Autodesk Fusion 360 part; units mm, degrees
note: some values were not read from the file. Chosen so that the rebuilt part matches the saved one: a direction. Set by a fixed rule: which sketch regions a step uses; which face or edge a step refers to.
(part 2 of 6)
  spline S261 degree 3 poles (85.6721, -57.6527) (85.6866, -57.6527) (85.6985, -57.6408) (85.6985, -57.6263) knots 0 0 0 0 1 1 1 1
  line L291 (85.6985, -57.6263) -> (85.6985, -56.0388)
  spline S262 degree 3 poles (85.6985, -56.0388) (85.6985, -56.0242) (85.6866, -56.0123) (85.6721, -56.0123) knots 0 0 0 0 1 1 1 1
  line L292 (85.6721, -56.0123) -> (84.9048, -56.0123)
  spline S263 degree 3 poles (84.9048, -56.0123) (84.8783, -56.0123) (84.9048, -56.0388) (84.9048, -56.0123) knots 0 0 0 0 1 1 1 1
  line L293 (84.9048, -56.0123) -> (84.9048, -54.4777)
  spline S264 degree 3 poles (84.9048, -54.4777) (84.9048, -54.4513) (84.8783, -54.4777) (84.9048, -54.4777) knots 0 0 0 0 1 1 1 1
  line L294 (84.9048, -54.4777) -> (85.6721, -54.4777)
  spline S265 degree 3 poles (85.6721, -54.4777) (85.6866, -54.4777) (85.6985, -54.4658) (85.6985, -54.4513) knots 0 0 0 0 1 1 1 1
  line L295 (85.6985, -54.4513) -> (85.6985, -52.8638)
  spline S266 degree 3 poles (85.6985, -52.8638) (85.6985, -52.8492) (85.6866, -52.8373) (85.6721, -52.8373) knots 0 0 0 0 1 1 1 1
  line L296 (85.6721, -52.8373) -> (84.9048, -52.8373)
  spline S267 degree 3 poles (84.9048, -52.8373) (84.8783, -52.8373) (84.9048, -52.8638) (84.9048, -52.8373) knots 0 0 0 0 1 1 1 1
  line L297 (84.9048, -52.8373) -> (84.9048, -51.3027)
  spline S268 degree 3 poles (84.9048, -51.3027) (84.9048, -51.2763) (84.8783, -51.3027) (84.9048, -51.3027) knots 0 0 0 0 1 1 1 1
  line L298 (84.9048, -51.3027) -> (85.6721, -51.3027)
  spline S269 degree 3 poles (85.6721, -51.3027) (85.6866, -51.3027) (85.6985, -51.2908) (85.6985, -51.2763) knots 0 0 0 0 1 1 1 1
  line L299 (85.6985, -51.2763) -> (85.6985, -49.6888)
  spline S270 degree 3 poles (85.6985, -49.6888) (85.6985, -49.6742) (85.6866, -49.6623) (85.6721, -49.6623) knots 0 0 0 0 1 1 1 1
  line L300 (85.6721, -49.6623) -> (84.9048, -49.6623)
  spline S271 degree 3 poles (84.9048, -49.6623) (84.8783, -49.6623) (84.9048, -49.6888) (84.9048, -49.6623) knots 0 0 0 0 1 1 1 1
  line L301 (84.9048, -49.6623) -> (84.9048, -48.1277)
  spline S272 degree 3 poles (84.9048, -48.1277) (84.9048, -48.1013) (84.8783, -48.1277) (84.9048, -48.1277) knots 0 0 0 0 1 1 1 1
  line L302 (84.9048, -48.1277) -> (85.6721, -48.1277)
  spline S273 degree 3 poles (85.6721, -48.1277) (85.6866, -48.1277) (85.6985, -48.1158) (85.6985, -48.1013) knots 0 0 0 0 1 1 1 1
  line L303 (85.6985, -48.1013) -> (85.6985, -46.5138)
  spline S274 degree 3 poles (85.6985, -46.5138) (85.6985, -46.4992) (85.6866, -46.4873) (85.6721, -46.4873) knots 0 0 0 0 1 1 1 1
  line L304 (85.6721, -46.4873) -> (84.9048, -46.4873)
  spline S275 degree 3 poles (84.9048, -46.4873) (84.8783, -46.4873) (84.9048, -46.5138) (84.9048, -46.4873) knots 0 0 0 0 1 1 1 1
  line L305 (84.9048, -46.4873) -> (84.9048, -44.9527)
  spline S276 degree 3 poles (84.9048, -44.9527) (84.9048, -44.9263) (84.8783, -44.9527) (84.9048, -44.9527) knots 0 0 0 0 1 1 1 1
  line L306 (84.9048, -44.9527) -> (85.6721, -44.9527)
  spline S277 degree 3 poles (85.6721, -44.9527) (85.6866, -44.9527) (85.6985, -44.9408) (85.6985, -44.9263) knots 0 0 0 0 1 1 1 1
  line L307 (85.6985, -44.9263) -> (85.6985, -43.3388)
  spline S278 degree 3 poles (85.6985, -43.3388) (85.6985, -43.3242) (85.6866, -43.3123) (85.6721, -43.3123) knots 0 0 0 0 1 1 1 1
  line L308 (85.6721, -43.3123) -> (84.9048, -43.3123)
  spline S279 degree 3 poles (84.9048, -43.3123) (84.8783, -43.3123) (84.9048, -43.3388) (84.9048, -43.3123) knots 0 0 0 0 1 1 1 1
  line L309 (84.9048, -43.3123) -> (84.9048, -42.5715)
  spline S280 degree 3 poles (84.9048, -42.5715) (84.9048, -42.545) (84.8783, -42.5715) (84.9048, -42.5715) knots 0 0 0 0 1 1 1 1
  line L310 (84.9048, -42.5715) -> (85.6721, -42.5715)
  spline S281 degree 3 poles (85.6721, -42.5715) (85.6866, -42.5715) (85.6985, -42.5596) (85.6985, -42.545) knots 0 0 0 0 1 1 1 1
  spline S282 degree 3 poles (85.6985, -42.545) (85.6985, -40.5432) (85.1718, -38.5768) (84.1708, -36.8432) knots 0 0 0 0 1 1 1 1
  spline S283 degree 3 poles (84.1708, -36.8432) (83.1699, -35.1097) (81.7303, -33.6701) (79.9968, -32.6692) knots 0 0 0 0 1 1 1 1
  spline S284 degree 3 poles (79.9968, -32.6692) (78.2632, -31.6682) (76.2968, -31.1415) (74.295, -31.1415) knots 0 0 0 0 1 1 1 1
  line L311 (74.295, -31.1415) -> (45.1908, -31.1415)
  spline S285 degree 3 poles (45.1908, -31.1415) (45.1763, -31.1415) (45.1644, -31.1534) (45.1644, -31.1679) knots 0 0 0 0 1 1 1 1
  line L312 (45.1644, -31.1679) -> (45.1644, -31.9617)
  line L313 (45.1644, -31.9617) -> (45.1644, -33.2581)
  spline S286 degree 3 poles (45.1644, -33.2581) (45.1644, -33.2846) (45.1908, -33.2581) (45.1644, -33.2581) knots 0 0 0 0 1 1 1 1
  line L314 (45.1644, -33.2581) -> (44.3971, -33.2581)
  spline S287 degree 3 poles (44.3971, -33.2581) (44.3825, -33.2581) (44.3706, -33.27) (44.3706, -33.2846) knots 0 0 0 0 1 1 1 1
  line L315 (44.3706, -33.2846) -> (44.3706, -34.8721)
  spline S288 degree 3 poles (44.3706, -34.8721) (44.3706, -34.8866) (44.3825, -34.8985) (44.3971, -34.8985) knots 0 0 0 0 1 1 1 1
  line L316 (44.3971, -34.8985) -> (45.1644, -34.8985)
  spline S289 degree 3 poles (45.1644, -34.8985) (45.1908, -34.8985) (45.1644, -34.8721) (45.1644, -34.8985) knots 0 0 0 0 1 1 1 1
  line L317 (45.1644, -34.8985) -> (45.1644, -36.4331)
  spline S290 degree 3 poles (45.1644, -36.4331) (45.1644, -36.4596) (45.1908, -36.4331) (45.1644, -36.4331) knots 0 0 0 0 1 1 1 1
  line L318 (45.1644, -36.4331) -> (44.3971, -36.4331)
  spline S291 degree 3 poles (44.3971, -36.4331) (44.3825, -36.4331) (44.3706, -36.445) (44.3706, -36.4596) knots 0 0 0 0 1 1 1 1
  line L319 (44.3706, -36.4596) -> (44.3706, -38.0471)
  spline S292 degree 3 poles (44.3706, -38.0471) (44.3706, -38.0616) (44.3825, -38.0735) (44.3971, -38.0735) knots 0 0 0 0 1 1 1 1
  line L320 (44.3971, -38.0735) -> (45.1644, -38.0735)
  spline S293 degree 3 poles (45.1644, -38.0735) (45.1908, -38.0735) (45.1644, -38.0471) (45.1644, -38.0735) knots 0 0 0 0 1 1 1 1
  line L321 (45.1644, -38.0735) -> (45.1644, -39.6081)
  spline S294 degree 3 poles (45.1644, -39.6081) (45.1644, -39.6346) (45.1908, -39.6081) (45.1644, -39.6081) knots 0 0 0 0 1 1 1 1
  line L322 (45.1644, -39.6081) -> (44.3971, -39.6081)
  spline S295 degree 3 poles (44.3971, -39.6081) (44.3825, -39.6081) (44.3706, -39.62) (44.3706, -39.6346) knots 0 0 0 0 1 1 1 1
  line L323 (44.3706, -39.6346) -> (44.3706, -41.2221)
  spline S296 degree 3 poles (44.3706, -41.2221) (44.3706, -41.2366) (44.3825, -41.2485) (44.3971, -41.2485) knots 0 0 0 0 1 1 1 1
  line L324 (44.3971, -41.2485) -> (45.1644, -41.2485)
  spline S297 degree 3 poles (45.1644, -41.2485) (45.1908, -41.2485) (45.1644, -41.2221) (45.1644, -41.2485) knots 0 0 0 0 1 1 1 1
  line L325 (45.1644, -41.2485) -> (45.1644, -42.7831)
  spline S298 degree 3 poles (45.1644, -42.7831) (45.1644, -42.8096) (45.1908, -42.7831) (45.1644, -42.7831) knots 0 0 0 0 1 1 1 1
  line L326 (45.1644, -42.7831) -> (44.3971, -42.7831)
  spline S299 degree 3 poles (44.3971, -42.7831) (44.3825, -42.7831) (44.3706, -42.795) (44.3706, -42.8096) knots 0 0 0 0 1 1 1 1
  line L327 (44.3706, -42.8096) -> (44.3706, -44.3971)
  spline S300 degree 3 poles (44.3706, -44.3971) (44.3706, -44.4116) (44.3825, -44.4235) (44.3971, -44.4235) knots 0 0 0 0 1 1 1 1
  line L328 (44.3971, -44.4235) -> (45.1644, -44.4235)
  spline S301 degree 3 poles (45.1644, -44.4235) (45.1908, -44.4235) (45.1644, -44.3971) (45.1644, -44.4235) knots 0 0 0 0 1 1 1 1
  line L329 (45.1644, -44.4235) -> (45.1644, -45.9581)
  spline S302 degree 3 poles (45.1644, -45.9581) (45.1644, -45.9846) (45.1908, -45.9581) (45.1644, -45.9581) knots 0 0 0 0 1 1 1 1
  line L330 (45.1644, -45.9581) -> (44.3971, -45.9581)
  spline S303 degree 3 poles (44.3971, -45.9581) (44.3825, -45.9581) (44.3706, -45.97) (44.3706, -45.9846) knots 0 0 0 0 1 1 1 1
  line L331 (44.3706, -45.9846) -> (44.3706, -47.5721)
  spline S304 degree 3 poles (44.3706, -47.5721) (44.3706, -47.5866) (44.3825, -47.5985) (44.3971, -47.5985) knots 0 0 0 0 1 1 1 1
  line L332 (44.3971, -47.5985) -> (45.1644, -47.5985)
  spline S305 degree 3 poles (45.1644, -47.5985) (45.1908, -47.5985) (45.1644, -47.5721) (45.1644, -47.5985) knots 0 0 0 0 1 1 1 1
  line L333 (45.1644, -47.5985) -> (45.1644, -49.1331)
  spline S306 degree 3 poles (45.1644, -49.1331) (45.1644, -49.1596) (45.1908, -49.1331) (45.1644, -49.1331) knots 0 0 0 0 1 1 1 1
  line L334 (45.1644, -49.1331) -> (44.3971, -49.1331)
  spline S307 degree 3 poles (44.3971, -49.1331) (44.3825, -49.1331) (44.3706, -49.145) (44.3706, -49.1596) knots 0 0 0 0 1 1 1 1
  line L335 (44.3706, -49.1596) -> (44.3706, -50.7471)
  spline S308 degree 3 poles (44.3706, -50.7471) (44.3706, -50.7616) (44.3825, -50.7735) (44.3971, -50.7735) knots 0 0 0 0 1 1 1 1
  line L336 (44.3971, -50.7735) -> (45.1644, -50.7735)
  spline S309 degree 3 poles (45.1644, -50.7735) (45.1908, -50.7735) (45.1644, -50.7471) (45.1644, -50.7735) knots 0 0 0 0 1 1 1 1
  line L337 (45.1644, -50.7735) -> (45.1644, -52.3081)
  spline S310 degree 3 poles (45.1644, -52.3081) (45.1644, -52.3346) (45.1908, -52.3081) (45.1644, -52.3081) knots 0 0 0 0 1 1 1 1
  line L338 (45.1644, -52.3081) -> (44.3971, -52.3081)
  spline S311 degree 3 poles (44.3971, -52.3081) (44.3825, -52.3081) (44.3706, -52.32) (44.3706, -52.3346) knots 0 0 0 0 1 1 1 1
  line L339 (44.3706, -52.3346) -> (44.3706, -53.9221)
  spline S312 degree 3 poles (44.3706, -53.9221) (44.3706, -53.9366) (44.3825, -53.9485) (44.3971, -53.9485) knots 0 0 0 0 1 1 1 1
  line L340 (44.3971, -53.9485) -> (45.1644, -53.9485)
  spline S313 degree 3 poles (45.1644, -53.9485) (45.1908, -53.9485) (45.1644, -53.9221) (45.1644, -53.9485) knots 0 0 0 0 1 1 1 1
  line L341 (45.1644, -53.9485) -> (45.1644, -55.4831)
  spline S314 degree 3 poles (45.1644, -55.4831) (45.1644, -55.5096) (45.1908, -55.4831) (45.1644, -55.4831) knots 0 0 0 0 1 1 1 1
  line L342 (45.1644, -55.4831) -> (44.3971, -55.4831)
  spline S315 degree 3 poles (44.3971, -55.4831) (44.3825, -55.4831) (44.3706, -55.495) (44.3706, -55.5096) knots 0 0 0 0 1 1 1 1
  line L343 (44.3706, -55.5096) -> (44.3706, -57.0971)
  spline S316 degree 3 poles (44.3706, -57.0971) (44.3706, -57.1116) (44.3825, -57.1235) (44.3971, -57.1235) knots 0 0 0 0 1 1 1 1
  line L344 (44.3971, -57.1235) -> (45.1644, -57.1235)
  spline S317 degree 3 poles (45.1644, -57.1235) (45.1908, -57.1235) (45.1644, -57.0971) (45.1644, -57.1235) knots 0 0 0 0 1 1 1 1
  line L345 (45.1644, -57.1235) -> (45.1644, -58.42)
  line L346 (86.9156, -58.4465) -> (88.2121, -58.4465)
  spline S318 degree 3 poles (88.2121, -58.4465) (88.2385, -58.4465) (88.2121, -58.42) (88.2121, -58.4465) knots 0 0 0 0 1 1 1 1
  line L347 (88.2121, -58.4465) -> (88.2121, -59.2138)
  spline S319 degree 3 poles (88.2121, -59.2138) (88.2121, -59.2283) (88.224, -59.2402) (88.2385, -59.2402) knots 0 0 0 0 1 1 1 1
  line L348 (88.2385, -59.2402) -> (89.826, -59.2402)
  spline S320 degree 3 poles (89.826, -59.2402) (89.8406, -59.2402) (89.8525, -59.2283) (89.8525, -59.2138) knots 0 0 0 0 1 1 1 1
  line L349 (89.8525, -59.2138) -> (89.8525, -58.4465)
  spline S321 degree 3 poles (89.8525, -58.4465) (89.8525, -58.42) (89.826, -58.4465) (89.8525, -58.4465) knots 0 0 0 0 1 1 1 1
  line L350 (89.8525, -58.4465) -> (91.3871, -58.4465)
  spline S322 degree 3 poles (91.3871, -58.4465) (91.4135, -58.4465) (91.3871, -58.42) (91.3871, -58.4465) knots 0 0 0 0 1 1 1 1
  line L351 (91.3871, -58.4465) -> (91.3871, -59.2138)
  spline S323 degree 3 poles (91.3871, -59.2138) (91.3871, -59.2283) (91.399, -59.2402) (91.4135, -59.2402) knots 0 0 0 0 1 1 1 1
  line L352 (91.4135, -59.2402) -> (93.001, -59.2402)
  spline S324 degree 3 poles (93.001, -59.2402) (93.0156, -59.2402) (93.0275, -59.2283) (93.0275, -59.2138) knots 0 0 0 0 1 1 1 1
  line L353 (93.0275, -59.2138) -> (93.0275, -58.4465)
  spline S325 degree 3 poles (93.0275, -58.4465) (93.0275, -58.42) (93.001, -58.4465) (93.0275, -58.4465) knots 0 0 0 0 1 1 1 1
  line L354 (93.0275, -58.4465) -> (94.5621, -58.4465)
  spline S326 degree 3 poles (94.5621, -58.4465) (94.5885, -58.4465) (94.5621, -58.42) (94.5621, -58.4465) knots 0 0 0 0 1 1 1 1
  line L355 (94.5621, -58.4465) -> (94.5621, -59.2138)
  spline S327 degree 3 poles (94.5621, -59.2138) (94.5621, -59.2283) (94.574, -59.2402) (94.5885, -59.2402) knots 0 0 0 0 1 1 1 1
  line L356 (94.5885, -59.2402) -> (96.176, -59.2402)
  spline S328 degree 3 poles (96.176, -59.2402) (96.1906, -59.2402) (96.2025, -59.2283) (96.2025, -59.2138) knots 0 0 0 0 1 1 1 1
  line L357 (96.2025, -59.2138) -> (96.2025, -58.4465)
  spline S329 degree 3 poles (96.2025, -58.4465) (96.2025, -58.42) (96.176, -58.4465) (96.2025, -58.4465) knots 0 0 0 0 1 1 1 1
  line L358 (96.2025, -58.4465) -> (97.7371, -58.4465)
  spline S330 degree 3 poles (97.7371, -58.4465) (97.7635, -58.4465) (97.7371, -58.42) (97.7371, -58.4465) knots 0 0 0 0 1 1 1 1
  line L359 (97.7371, -58.4465) -> (97.7371, -59.2138)
  spline S331 degree 3 poles (97.7371, -59.2138) (97.7371, -59.2283) (97.749, -59.2402) (97.7635, -59.2402) knots 0 0 0 0 1 1 1 1
  line L360 (97.7635, -59.2402) -> (99.351, -59.2402)
  spline S332 degree 3 poles (99.351, -59.2402) (99.3656, -59.2402) (99.3775, -59.2283) (99.3775, -59.2138) knots 0 0 0 0 1 1 1 1
  line L361 (99.3775, -59.2138) -> (99.3775, -58.4465)
  spline S333 degree 3 poles (99.3775, -58.4465) (99.3775, -58.42) (99.351, -58.4465) (99.3775, -58.4465) knots 0 0 0 0 1 1 1 1
  line L362 (99.3775, -58.4465) -> (100.9121, -58.4465)
  spline S334 degree 3 poles (100.9121, -58.4465) (100.9385, -58.4465) (100.9121, -58.42) (100.9121, -58.4465) knots 0 0 0 0 1 1 1 1
  line L363 (100.9121, -58.4465) -> (100.9121, -59.2138)
  spline S335 degree 3 poles (100.9121, -59.2138) (100.9121, -59.2283) (100.924, -59.2402) (100.9385, -59.2402) knots 0 0 0 0 1 1 1 1
  line L364 (100.9385, -59.2402) -> (102.526, -59.2402)
  spline S336 degree 3 poles (102.526, -59.2402) (102.5406, -59.2402) (102.5525, -59.2283) (102.5525, -59.2138) knots 0 0 0 0 1 1 1 1
  line L365 (102.5525, -59.2138) -> (102.5525, -58.4465)
  spline S337 degree 3 poles (102.5525, -58.4465) (102.5525, -58.42) (102.526, -58.4465) (102.5525, -58.4465) knots 0 0 0 0 1 1 1 1
  line L366 (102.5525, -58.4465) -> (104.0871, -58.4465)
  spline S338 degree 3 poles (104.0871, -58.4465) (104.1135, -58.4465) (104.0871, -58.42) (104.0871, -58.4465) knots 0 0 0 0 1 1 1 1
  line L367 (104.0871, -58.4465) -> (104.0871, -59.2138)
  spline S339 degree 3 poles (104.0871, -59.2138) (104.0871, -59.2283) (104.099, -59.2402) (104.1135, -59.2402) knots 0 0 0 0 1 1 1 1
  line L368 (104.1135, -59.2402) -> (105.701, -59.2402)
  spline S340 degree 3 poles (105.701, -59.2402) (105.7156, -59.2402) (105.7275, -59.2283) (105.7275, -59.2138) knots 0 0 0 0 1 1 1 1
  line L369 (105.7275, -59.2138) -> (105.7275, -58.4465)
  spline S341 degree 3 poles (105.7275, -58.4465) (105.7275, -58.42) (105.701, -58.4465) (105.7275, -58.4465) knots 0 0 0 0 1 1 1 1
  line L370 (105.7275, -58.4465) -> (107.2621, -58.4465)
  spline S342 degree 3 poles (107.2621, -58.4465) (107.2885, -58.4465) (107.2621, -58.42) (107.2621, -58.4465) knots 0 0 0 0 1 1 1 1
  line L371 (107.2621, -58.4465) -> (107.2621, -59.2138)
  spline S343 degree 3 poles (107.2621, -59.2138) (107.2621, -59.2283) (107.274, -59.2402) (107.2885, -59.2402) knots 0 0 0 0 1 1 1 1
  line L372 (107.2885, -59.2402) -> (108.876, -59.2402)
  spline S344 degree 3 poles (108.876, -59.2402) (108.8906, -59.2402) (108.9025, -59.2283) (108.9025, -59.2138) knots 0 0 0 0 1 1 1 1
  line L373 (108.9025, -59.2138) -> (108.9025, -58.4465)
  spline S345 degree 3 poles (108.9025, -58.4465) (108.9025, -58.42) (108.876, -58.4465) (108.9025, -58.4465) knots 0 0 0 0 1 1 1 1
  line L374 (108.9025, -58.4465) -> (110.4371, -58.4465)
  spline S346 degree 3 poles (110.4371, -58.4465) (110.4635, -58.4465) (110.4371, -58.42) (110.4371, -58.4465) knots 0 0 0 0 1 1 1 1
  line L375 (110.4371, -58.4465) -> (110.4371, -59.2138)
  spline S347 degree 3 poles (110.4371, -59.2138) (110.4371, -59.2283) (110.449, -59.2402) (110.4635, -59.2402) knots 0 0 0 0 1 1 1 1
  line L376 (110.4635, -59.2402) -> (112.051, -59.2402)
  spline S348 degree 3 poles (112.051, -59.2402) (112.0656, -59.2402) (112.0775, -59.2283) (112.0775, -59.2138) knots 0 0 0 0 1 1 1 1
  line L377 (112.0775, -59.2138) -> (112.0775, -58.4465)
  spline S349 degree 3 poles (112.0775, -58.4465) (112.0775, -58.42) (112.051, -58.4465) (112.0775, -58.4465) knots 0 0 0 0 1 1 1 1
  line L378 (112.0775, -58.4465) -> (113.374, -58.4465)
  line L379 (113.374, -58.4465) -> (114.1677, -58.4465)
  spline S350 degree 3 poles (114.1677, -58.4465) (114.1823, -58.4465) (114.1942, -58.4346) (114.1942, -58.42) knots 0 0 0 0 1 1 1 1
  line L380 (114.1942, -58.42) -> (114.1942, -57.0971)
  spline S351 degree 3 poles (114.1942, -57.0971) (114.1942, -57.0825) (114.1823, -57.0706) (114.1677, -57.0706) knots 0 0 0 0 1 1 1 1
  line L381 (114.1677, -57.0706) -> (113.4004, -57.0706)
  spline S352 degree 3 poles (113.4004, -57.0706) (113.374, -57.0706) (113.4004, -57.0971) (113.4004, -57.0706) knots 0 0 0 0 1 1 1 1
  line L382 (113.4004, -57.0706) -> (113.4004, -55.536)
  spline S353 degree 3 poles (113.4004, -55.536) (113.4004, -55.5096) (113.374, -55.536) (113.4004, -55.536) knots 0 0 0 0 1 1 1 1
  line L383 (113.4004, -55.536) -> (114.1677, -55.536)
  spline S354 degree 3 poles (114.1677, -55.536) (114.1823, -55.536) (114.1942, -55.5241) (114.1942, -55.5096) knots 0 0 0 0 1 1 1 1
  line L384 (114.1942, -55.5096) -> (114.1942, -53.9221)
  spline S355 degree 3 poles (114.1942, -53.9221) (114.1942, -53.9075) (114.1823, -53.8956) (114.1677, -53.8956) knots 0 0 0 0 1 1 1 1
  line L385 (114.1677, -53.8956) -> (113.4004, -53.8956)
  spline S356 degree 3 poles (113.4004, -53.8956) (113.374, -53.8956) (113.4004, -53.9221) (113.4004, -53.8956) knots 0 0 0 0 1 1 1 1
  line L386 (113.4004, -53.8956) -> (113.4004, -52.361)
  spline S357 degree 3 poles (113.4004, -52.361) (113.4004, -52.3346) (113.374, -52.361) (113.4004, -52.361) knots 0 0 0 0 1 1 1 1
  line L387 (113.4004, -52.361) -> (114.1677, -52.361)
  spline S358 degree 3 poles (114.1677, -52.361) (114.1823, -52.361) (114.1942, -52.3491) (114.1942, -52.3346) knots 0 0 0 0 1 1 1 1
  line L388 (114.1942, -52.3346) -> (114.1942, -50.7471)
  spline S359 degree 3 poles (114.1942, -50.7471) (114.1942, -50.7325) (114.1823, -50.7206) (114.1677, -50.7206) knots 0 0 0 0 1 1 1 1
  line L389 (114.1677, -50.7206) -> (113.4004, -50.7206)
  spline S360 degree 3 poles (113.4004, -50.7206) (113.374, -50.7206) (113.4004, -50.7471) (113.4004, -50.7206) knots 0 0 0 0 1 1 1 1
  line L390 (113.4004, -50.7206) -> (113.4004, -49.186)
  spline S361 degree 3 poles (113.4004, -49.186) (113.4004, -49.1596) (113.374, -49.186) (113.4004, -49.186) knots 0 0 0 0 1 1 1 1
  line L391 (113.4004, -49.186) -> (114.1677, -49.186)
  spline S362 degree 3 poles (114.1677, -49.186) (114.1823, -49.186) (114.1942, -49.1741) (114.1942, -49.1596) knots 0 0 0 0 1 1 1 1
  line L392 (114.1942, -49.1596) -> (114.1942, -47.5721)
  spline S363 degree 3 poles (114.1942, -47.5721) (114.1942, -47.5575) (114.1823, -47.5456) (114.1677, -47.5456) knots 0 0 0 0 1 1 1 1
  line L393 (114.1677, -47.5456) -> (113.4004, -47.5456)
  spline S364 degree 3 poles (113.4004, -47.5456) (113.374, -47.5456) (113.4004, -47.5721) (113.4004, -47.5456) knots 0 0 0 0 1 1 1 1
  line L394 (113.4004, -47.5456) -> (113.4004, -46.011)
  spline S365 degree 3 poles (113.4004, -46.011) (113.4004, -45.9846) (113.374, -46.011) (113.4004, -46.011) knots 0 0 0 0 1 1 1 1
  line L395 (113.4004, -46.011) -> (114.1677, -46.011)
  spline S366 degree 3 poles (114.1677, -46.011) (114.1823, -46.011) (114.1942, -45.9991) (114.1942, -45.9846) knots 0 0 0 0 1 1 1 1
  line L396 (114.1942, -45.9846) -> (114.1942, -44.3971)
  spline S367 degree 3 poles (114.1942, -44.3971) (114.1942, -44.3825) (114.1823, -44.3706) (114.1677, -44.3706) knots 0 0 0 0 1 1 1 1
  line L397 (114.1677, -44.3706) -> (113.4004, -44.3706)
  spline S368 degree 3 poles (113.4004, -44.3706) (113.374, -44.3706) (113.4004, -44.3971) (113.4004, -44.3706) knots 0 0 0 0 1 1 1 1
  line L398 (113.4004, -44.3706) -> (113.4004, -42.836)
  spline S369 degree 3 poles (113.4004, -42.836) (113.4004, -42.8096) (113.374, -42.836) (113.4004, -42.836) knots 0 0 0 0 1 1 1 1
  line L399 (113.4004, -42.836) -> (114.1677, -42.836)
  spline S370 degree 3 poles (114.1677, -42.836) (114.1823, -42.836) (114.1942, -42.8241) (114.1942, -42.8096) knots 0 0 0 0 1 1 1 1
  line L400 (114.1942, -42.8096) -> (114.1942, -41.2221)
  spline S371 degree 3 poles (114.1942, -41.2221) (114.1942, -41.2075) (114.1823, -41.1956) (114.1677, -41.1956) knots 0 0 0 0 1 1 1 1
  line L401 (114.1677, -41.1956) -> (113.4004, -41.1956)
  spline S372 degree 3 poles (113.4004, -41.1956) (113.374, -41.1956) (113.4004, -41.2221) (113.4004, -41.1956) knots 0 0 0 0 1 1 1 1
  line L402 (113.4004, -41.1956) -> (113.4004, -39.661)
  spline S373 degree 3 poles (113.4004, -39.661) (113.4004, -39.6346) (113.374, -39.661) (113.4004, -39.661) knots 0 0 0 0 1 1 1 1
  line L403 (113.4004, -39.661) -> (114.1677, -39.661)
  spline S374 degree 3 poles (114.1677, -39.661) (114.1823, -39.661) (114.1942, -39.6491) (114.1942, -39.6346) knots 0 0 0 0 1 1 1 1
  line L404 (114.1942, -39.6346) -> (114.1942, -38.0471)
  spline S375 degree 3 poles (114.1942, -38.0471) (114.1942, -38.0325) (114.1823, -38.0206) (114.1677, -38.0206) knots 0 0 0 0 1 1 1 1
  line L405 (114.1677, -38.0206) -> (113.4004, -38.0206)
  spline S376 degree 3 poles (113.4004, -38.0206) (113.374, -38.0206) (113.4004, -38.0471) (113.4004, -38.0206) knots 0 0 0 0 1 1 1 1
  line L406 (113.4004, -38.0206) -> (113.4004, -36.486)
  spline S377 degree 3 poles (113.4004, -36.486) (113.4004, -36.4596) (113.374, -36.486) (113.4004, -36.486) knots 0 0 0 0 1 1 1 1
  line L407 (113.4004, -36.486) -> (114.1677, -36.486)
  spline S378 degree 3 poles (114.1677, -36.486) (114.1823, -36.486) (114.1942, -36.4741) (114.1942, -36.4596) knots 0 0 0 0 1 1 1 1
  line L408 (114.1942, -36.4596) -> (114.1942, -34.8721)
  spline S379 degree 3 poles (114.1942, -34.8721) (114.1942, -34.8575) (114.1823, -34.8456) (114.1677, -34.8456) knots 0 0 0 0 1 1 1 1
  line L409 (114.1677, -34.8456) -> (113.4004, -34.8456)
  spline S380 degree 3 poles (113.4004, -34.8456) (113.374, -34.8456) (113.4004, -34.8721) (113.4004, -34.8456) knots 0 0 0 0 1 1 1 1
  line L410 (113.4004, -34.8456) -> (113.4004, -33.311)
  spline S381 degree 3 poles (113.4004, -33.311) (113.4004, -33.2846) (113.374, -33.311) (113.4004, -33.311) knots 0 0 0 0 1 1 1 1
  line L411 (113.4004, -33.311) -> (114.1677, -33.311)
  spline S382 degree 3 poles (114.1677, -33.311) (114.1823, -33.311) (114.1942, -33.2991) (114.1942, -33.2846) knots 0 0 0 0 1 1 1 1
  line L412 (114.1942, -33.2846) -> (114.1942, -31.9617)
  line L413 (114.1942, -31.9617) -> (114.1942, -31.1679)
  spline S383 degree 3 poles (114.1942, -31.1679) (114.1942, -31.1534) (114.1823, -31.1415) (114.1677, -31.1415) knots 0 0 0 0 1 1 1 1
  line L414 (114.1677, -31.1415) -> (113.374, -31.1415)
  line L415 (113.374, -31.1415) -> (86.9156, -31.1415)
  line L416 (86.9156, -31.1415) -> (86.1219, -31.1415)
  spline S384 degree 3 poles (86.1219, -31.1415) (86.1073, -31.1415) (86.0954, -31.1534) (86.0954, -31.1679) knots 0 0 0 0 1 1 1 1
  line L417 (86.0954, -31.1679) -> (86.0954, -31.9617)
  line L418 (86.0954, -31.9617) -> (86.0954, -33.2846)
  spline S385 degree 3 poles (86.0954, -33.2846) (86.0954, -33.2991) (86.1073, -33.311) (86.1219, -33.311) knots 0 0 0 0 1 1 1 1
  line L419 (86.1219, -33.311) -> (86.8892, -33.311)
  spline S386 degree 3 poles (86.8892, -33.311) (86.9156, -33.311) (86.8892, -33.2846) (86.8892, -33.311) knots 0 0 0 0 1 1 1 1
  line L420 (86.8892, -33.311) -> (86.8892, -34.8456)
  spline S387 degree 3 poles (86.8892, -34.8456) (86.8892, -34.8721) (86.9156, -34.8456) (86.8892, -34.8456) knots 0 0 0 0 1 1 1 1
  line L421 (86.8892, -34.8456) -> (86.1219, -34.8456)
  spline S388 degree 3 poles (86.1219, -34.8456) (86.1073, -34.8456) (86.0954, -34.8575) (86.0954, -34.8721) knots 0 0 0 0 1 1 1 1
  line L422 (86.0954, -34.8721) -> (86.0954, -36.4596)
  spline S389 degree 3 poles (86.0954, -36.4596) (86.0954, -36.4741) (86.1073, -36.486) (86.1219, -36.486) knots 0 0 0 0 1 1 1 1
  line L423 (86.1219, -36.486) -> (86.8892, -36.486)
  spline S390 degree 3 poles (86.8892, -36.486) (86.9156, -36.486) (86.8892, -36.4596) (86.8892, -36.486) knots 0 0 0 0 1 1 1 1
  line L424 (86.8892, -36.486) -> (86.8892, -38.0206)
  spline S391 degree 3 poles (86.8892, -38.0206) (86.8892, -38.0471) (86.9156, -38.0206) (86.8892, -38.0206) knots 0 0 0 0 1 1 1 1
  line L425 (86.8892, -38.0206) -> (86.1219, -38.0206)
  spline S392 degree 3 poles (86.1219, -38.0206) (86.1073, -38.0206) (86.0954, -38.0325) (86.0954, -38.0471) knots 0 0 0 0 1 1 1 1
  line L426 (86.0954, -38.0471) -> (86.0954, -39.6346)
  spline S393 degree 3 poles (86.0954, -39.6346) (86.0954, -39.6491) (86.1073, -39.661) (86.1219, -39.661) knots 0 0 0 0 1 1 1 1
  line L427 (86.1219, -39.661) -> (86.8892, -39.661)
  spline S394 degree 3 poles (86.8892, -39.661) (86.9156, -39.661) (86.8892, -39.6346) (86.8892, -39.661) knots 0 0 0 0 1 1 1 1
  line L428 (86.8892, -39.661) -> (86.8892, -41.1956)
  spline S395 degree 3 poles (86.8892, -41.1956) (86.8892, -41.2221) (86.9156, -41.1956) (86.8892, -41.1956) knots 0 0 0 0 1 1 1 1
  line L429 (86.8892, -41.1956) -> (86.1219, -41.1956)
  spline S396 degree 3 poles (86.1219, -41.1956) (86.1073, -41.1956) (86.0954, -41.2075) (86.0954, -41.2221) knots 0 0 0 0 1 1 1 1
  line L430 (86.0954, -41.2221) -> (86.0954, -42.8096)
  spline S397 degree 3 poles (86.0954, -42.8096) (86.0954, -42.8241) (86.1073, -42.836) (86.1219, -42.836) knots 0 0 0 0 1 1 1 1
  line L431 (86.1219, -42.836) -> (86.8892, -42.836)
  spline S398 degree 3 poles (86.8892, -42.836) (86.9156, -42.836) (86.8892, -42.8096) (86.8892, -42.836) knots 0 0 0 0 1 1 1 1
  line L432 (86.8892, -42.836) -> (86.8892, -44.3706)
  spline S399 degree 3 poles (86.8892, -44.3706) (86.8892, -44.3971) (86.9156, -44.3706) (86.8892, -44.3706) knots 0 0 0 0 1 1 1 1
  line L433 (86.8892, -44.3706) -> (86.1219, -44.3706)
  spline S400 degree 3 poles (86.1219, -44.3706) (86.1073, -44.3706) (86.0954, -44.3825) (86.0954, -44.3971) knots 0 0 0 0 1 1 1 1
  line L434 (86.0954, -44.3971) -> (86.0954, -45.9846)
  spline S401 degree 3 poles (86.0954, -45.9846) (86.0954, -45.9991) (86.1073, -46.011) (86.1219, -46.011) knots 0 0 0 0 1 1 1 1
  line L435 (86.1219, -46.011) -> (86.8892, -46.011)
  spline S402 degree 3 poles (86.8892, -46.011) (86.9156, -46.011) (86.8892, -45.9846) (86.8892, -46.011) knots 0 0 0 0 1 1 1 1
  line L436 (86.8892, -46.011) -> (86.8892, -47.5456)
  spline S403 degree 3 poles (86.8892, -47.5456) (86.8892, -47.5721) (86.9156, -47.5456) (86.8892, -47.5456) knots 0 0 0 0 1 1 1 1
  line L437 (86.8892, -47.5456) -> (86.1219, -47.5456)
  spline S404 degree 3 poles (86.1219, -47.5456) (86.1073, -47.5456) (86.0954, -47.5575) (86.0954, -47.5721) knots 0 0 0 0 1 1 1 1
  line L438 (86.0954, -47.5721) -> (86.0954, -49.1596)
  spline S405 degree 3 poles (86.0954, -49.1596) (86.0954, -49.1741) (86.1073, -49.186) (86.1219, -49.186) knots 0 0 0 0 1 1 1 1
  line L439 (86.1219, -49.186) -> (86.8892, -49.186)
  spline S406 degree 3 poles (86.8892, -49.186) (86.9156, -49.186) (86.8892, -49.1596) (86.8892, -49.186) knots 0 0 0 0 1 1 1 1
  line L440 (86.8892, -49.186) -> (86.8892, -50.7206)
  spline S407 degree 3 poles (86.8892, -50.7206) (86.8892, -50.7471) (86.9156, -50.7206) (86.8892, -50.7206) knots 0 0 0 0 1 1 1 1
  line L441 (86.8892, -50.7206) -> (86.1219, -50.7206)
  spline S408 degree 3 poles (86.1219, -50.7206) (86.1073, -50.7206) (86.0954, -50.7325) (86.0954, -50.7471) knots 0 0 0 0 1 1 1 1
  line L442 (86.0954, -50.7471) -> (86.0954, -52.3346)
  spline S409 degree 3 poles (86.0954, -52.3346) (86.0954, -52.3491) (86.1073, -52.361) (86.1219, -52.361) knots 0 0 0 0 1 1 1 1
  line L443 (86.1219, -52.361) -> (86.8892, -52.361)
  spline S410 degree 3 poles (86.8892, -52.361) (86.9156, -52.361) (86.8892, -52.3346) (86.8892, -52.361) knots 0 0 0 0 1 1 1 1
  line L444 (86.8892, -52.361) -> (86.8892, -53.8956)
  spline S411 degree 3 poles (86.8892, -53.8956) (86.8892, -53.9221) (86.9156, -53.8956) (86.8892, -53.8956) knots 0 0 0 0 1 1 1 1
  line L445 (86.8892, -53.8956) -> (86.1219, -53.8956)
  spline S412 degree 3 poles (86.1219, -53.8956) (86.1073, -53.8956) (86.0954, -53.9075) (86.0954, -53.9221) knots 0 0 0 0 1 1 1 1
  line L446 (86.0954, -53.9221) -> (86.0954, -55.5096)
  spline S413 degree 3 poles (86.0954, -55.5096) (86.0954, -55.5241) (86.1073, -55.536) (86.1219, -55.536) knots 0 0 0 0 1 1 1 1
  line L447 (86.1219, -55.536) -> (86.8892, -55.536)
  spline S414 degree 3 poles (86.8892, -55.536) (86.9156, -55.536) (86.8892, -55.5096) (86.8892, -55.536) knots 0 0 0 0 1 1 1 1
  line L448 (86.8892, -55.536) -> (86.8892, -57.0706)
  spline S415 degree 3 poles (86.8892, -57.0706) (86.8892, -57.0971) (86.9156, -57.0706) (86.8892, -57.0706) knots 0 0 0 0 1 1 1 1
  line L449 (86.8892, -57.0706) -> (86.1219, -57.0706)
  spline S416 degree 3 poles (86.1219, -57.0706) (86.1073, -57.0706) (86.0954, -57.0825) (86.0954, -57.0971) knots 0 0 0 0 1 1 1 1
  line L450 (86.0954, -57.0971) -> (86.0954, -58.42)
  spline S417 degree 3 poles (86.0954, -58.42) (86.0954, -58.4346) (86.1073, -58.4465) (86.1219, -58.4465) knots 0 0 0 0 1 1 1 1
  line L451 (86.1219, -58.4465) -> (86.9156, -58.4465)
  line L452 (115.4113, -58.4465) -> (116.7077, -58.4465)
  spline S418 degree 3 poles (116.7077, -58.4465) (116.7342, -58.4465) (116.7077, -58.42) (116.7077, -58.4465) knots 0 0 0 0 1 1 1 1
  line L453 (116.7077, -58.4465) -> (116.7077, -59.2138)
  spline S419 degree 3 poles (116.7077, -59.2138) (116.7077, -59.2283) (116.7196, -59.2402) (116.7342, -59.2402) knots 0 0 0 0 1 1 1 1
  line L454 (116.7342, -59.2402) -> (118.3217, -59.2402)
  spline S420 degree 3 poles (118.3217, -59.2402) (118.3362, -59.2402) (118.3481, -59.2283) (118.3481, -59.2138) knots 0 0 0 0 1 1 1 1
  line L455 (118.3481, -59.2138) -> (118.3481, -58.4465)
  spline S421 degree 3 poles (118.3481, -58.4465) (118.3481, -58.42) (118.3217, -58.4465) (118.3481, -58.4465) knots 0 0 0 0 1 1 1 1
  line L456 (118.3481, -58.4465) -> (119.8827, -58.4465)
  spline S422 degree 3 poles (119.8827, -58.4465) (119.9092, -58.4465) (119.8827, -58.42) (119.8827, -58.4465) knots 0 0 0 0 1 1 1 1
  line L457 (119.8827, -58.4465) -> (119.8827, -59.2138)
  spline S423 degree 3 poles (119.8827, -59.2138) (119.8827, -59.2283) (119.8946, -59.2402) (119.9092, -59.2402) knots 0 0 0 0 1 1 1 1
  line L458 (119.9092, -59.2402) -> (121.4967, -59.2402)
  spline S424 degree 3 poles (121.4967, -59.2402) (121.5112, -59.2402) (121.5231, -59.2283) (121.5231, -59.2138) knots 0 0 0 0 1 1 1 1
  line L459 (121.5231, -59.2138) -> (121.5231, -58.4465)
  spline S425 degree 3 poles (121.5231, -58.4465) (121.5231, -58.42) (121.4967, -58.4465) (121.5231, -58.4465) knots 0 0 0 0 1 1 1 1
  line L460 (121.5231, -58.4465) -> (123.0577, -58.4465)
  spline S426 degree 3 poles (123.0577, -58.4465) (123.0842, -58.4465) (123.0577, -58.42) (123.0577, -58.4465) knots 0 0 0 0 1 1 1 1
  line L461 (123.0577, -58.4465) -> (123.0577, -59.2138)
  spline S427 degree 3 poles (123.0577, -59.2138) (123.0577, -59.2283) (123.0696, -59.2402) (123.0842, -59.2402) knots 0 0 0 0 1 1 1 1
  line L462 (123.0842, -59.2402) -> (124.6717, -59.2402)
  spline S428 degree 3 poles (124.6717, -59.2402) (124.6862, -59.2402) (124.6981, -59.2283) (124.6981, -59.2138) knots 0 0 0 0 1 1 1 1
  line L463 (124.6981, -59.2138) -> (124.6981, -58.4465)
  spline S429 degree 3 poles (124.6981, -58.4465) (124.6981, -58.42) (124.6717, -58.4465) (124.6981, -58.4465) knots 0 0 0 0 1 1 1 1
  line L464 (124.6981, -58.4465) -> (126.2327, -58.4465)
  spline S430 degree 3 poles (126.2327, -58.4465) (126.2592, -58.4465) (126.2327, -58.42) (126.2327, -58.4465) knots 0 0 0 0 1 1 1 1
  line L465 (126.2327, -58.4465) -> (126.2327, -59.2138)
  spline S431 degree 3 poles (126.2327, -59.2138) (126.2327, -59.2283) (126.2446, -59.2402) (126.2592, -59.2402) knots 0 0 0 0 1 1 1 1
  line L466 (126.2592, -59.2402) -> (127.8467, -59.2402)
  spline S432 degree 3 poles (127.8467, -59.2402) (127.8612, -59.2402) (127.8731, -59.2283) (127.8731, -59.2138) knots 0 0 0 0 1 1 1 1
  line L467 (127.8731, -59.2138) -> (127.8731, -58.4465)
  spline S433 degree 3 poles (127.8731, -58.4465) (127.8731, -58.42) (127.8467, -58.4465) (127.8731, -58.4465) knots 0 0 0 0 1 1 1 1
  line L468 (127.8731, -58.4465) -> (129.4077, -58.4465)
  spline S434 degree 3 poles (129.4077, -58.4465) (129.4342, -58.4465) (129.4077, -58.42) (129.4077, -58.4465) knots 0 0 0 0 1 1 1 1
  line L469 (129.4077, -58.4465) -> (129.4077, -59.2138)
  spline S435 degree 3 poles (129.4077, -59.2138) (129.4077, -59.2283) (129.4196, -59.2402) (129.4342, -59.2402) knots 0 0 0 0 1 1 1 1
  line L470 (129.4342, -59.2402) -> (131.0217, -59.2402)
  spline S436 degree 3 poles (131.0217, -59.2402) (131.0362, -59.2402) (131.0481, -59.2283) (131.0481, -59.2138) knots 0 0 0 0 1 1 1 1
  line L471 (131.0481, -59.2138) -> (131.0481, -58.4465)
  spline S437 degree 3 poles (131.0481, -58.4465) (131.0481, -58.42) (131.0217, -58.4465) (131.0481, -58.4465) knots 0 0 0 0 1 1 1 1
  line L472 (131.0481, -58.4465) -> (132.5827, -58.4465)
  spline S438 degree 3 poles (132.5827, -58.4465) (132.6092, -58.4465) (132.5827, -58.42) (132.5827, -58.4465) knots 0 0 0 0 1 1 1 1
  line L473 (132.5827, -58.4465) -> (132.5827, -59.2138)
  spline S439 degree 3 poles (132.5827, -59.2138) (132.5827, -59.2283) (132.5946, -59.2402) (132.6092, -59.2402) knots 0 0 0 0 1 1 1 1
  line L474 (132.6092, -59.2402) -> (134.1967, -59.2402)
  spline S440 degree 3 poles (134.1967, -59.2402) (134.2112, -59.2402) (134.2231, -59.2283) (134.2231, -59.2138) knots 0 0 0 0 1 1 1 1
  line L475 (134.2231, -59.2138) -> (134.2231, -58.4465)
  spline S441 degree 3 poles (134.2231, -58.4465) (134.2231, -58.42) (134.1967, -58.4465) (134.2231, -58.4465) knots 0 0 0 0 1 1 1 1
  line L476 (134.2231, -58.4465) -> (135.7577, -58.4465)
  spline S442 degree 3 poles (135.7577, -58.4465) (135.7842, -58.4465) (135.7577, -58.42) (135.7577, -58.4465) knots 0 0 0 0 1 1 1 1
  line L477 (135.7577, -58.4465) -> (135.7577, -59.2138)
  spline S443 degree 3 poles (135.7577, -59.2138) (135.7577, -59.2283) (135.7696, -59.2402) (135.7842, -59.2402) knots 0 0 0 0 1 1 1 1
  line L478 (135.7842, -59.2402) -> (137.3717, -59.2402)
  spline S444 degree 3 poles (137.3717, -59.2402) (137.3862, -59.2402) (137.3981, -59.2283) (137.3981, -59.2138) knots 0 0 0 0 1 1 1 1
  line L479 (137.3981, -59.2138) -> (137.3981, -58.4465)
  spline S445 degree 3 poles (137.3981, -58.4465) (137.3981, -58.42) (137.3717, -58.4465) (137.3981, -58.4465) knots 0 0 0 0 1 1 1 1
  line L480 (137.3981, -58.4465) -> (138.9327, -58.4465)
  spline S446 degree 3 poles (138.9327, -58.4465) (138.9592, -58.4465) (138.9327, -58.42) (138.9327, -58.4465) knots 0 0 0 0 1 1 1 1
  line L481 (138.9327, -58.4465) -> (138.9327, -59.2138)
  spline S447 degree 3 poles (138.9327, -59.2138) (138.9327, -59.2283) (138.9446, -59.2402) (138.9592, -59.2402) knots 0 0 0 0 1 1 1 1
  line L482 (138.9592, -59.2402) -> (140.5467, -59.2402)
  spline S448 degree 3 poles (140.5467, -59.2402) (140.5612, -59.2402) (140.5731, -59.2283) (140.5731, -59.2138) knots 0 0 0 0 1 1 1 1
  line L483 (140.5731, -59.2138) -> (140.5731, -58.4465)
  spline S449 degree 3 poles (140.5731, -58.4465) (140.5731, -58.42) (140.5467, -58.4465) (140.5731, -58.4465) knots 0 0 0 0 1 1 1 1
  line L484 (140.5731, -58.4465) -> (141.8696, -58.4465)
  line L485 (141.8696, -58.4465) -> (142.6633, -58.4465)
  spline S450 degree 3 poles (142.6633, -58.4465) (142.6779, -58.4465) (142.6898, -58.4346) (142.6898, -58.42) knots 0 0 0 0 1 1 1 1
  line L486 (142.6898, -58.42) -> (142.6898, -57.6263)
  spline S451 degree 3 poles (142.6898, -57.6263) (142.6898, -57.6117) (142.6779, -57.5998) (142.6633, -57.5998) knots 0 0 0 0 1 1 1 1
  line L487 (142.6633, -57.5998) -> (141.896, -57.5998)
  spline S452 degree 3 poles (141.896, -57.5998) (141.8696, -57.5998) (141.896, -57.6263) (141.896, -57.5998) knots 0 0 0 0 1 1 1 1
  line L488 (141.896, -57.5998) -> (141.896, -56.0652)
  spline S453 degree 3 poles (141.896, -56.0652) (141.896, -56.0388) (141.8696, -56.0652) (141.896, -56.0652) knots 0 0 0 0 1 1 1 1
  line L489 (141.896, -56.0652) -> (142.6633, -56.0652)
  spline S454 degree 3 poles (142.6633, -56.0652) (142.6779, -56.0652) (142.6898, -56.0533) (142.6898, -56.0388) knots 0 0 0 0 1 1 1 1
  line L490 (142.6898, -56.0388) -> (142.6898, -54.4513)
  spline S455 degree 3 poles (142.6898, -54.4513) (142.6898, -54.4367) (142.6779, -54.4248) (142.6633, -54.4248) knots 0 0 0 0 1 1 1 1
  line L491 (142.6633, -54.4248) -> (141.896, -54.4248)
  spline S456 degree 3 poles (141.896, -54.4248) (141.8696, -54.4248) (141.896, -54.4513) (141.896, -54.4248) knots 0 0 0 0 1 1 1 1
  line L492 (141.896, -54.4248) -> (141.896, -52.8902)
  spline S457 degree 3 poles (141.896, -52.8902) (141.896, -52.8638) (141.8696, -52.8902) (141.896, -52.8902) knots 0 0 0 0 1 1 1 1
  line L493 (141.896, -52.8902) -> (142.6633, -52.8902)
  spline S458 degree 3 poles (142.6633, -52.8902) (142.6779, -52.8902) (142.6898, -52.8783) (142.6898, -52.8638) knots 0 0 0 0 1 1 1 1
  line L494 (142.6898, -52.8638) -> (142.6898, -51.2763)
  spline S459 degree 3 poles (142.6898, -51.2763) (142.6898, -51.2617) (142.6779, -51.2498) (142.6633, -51.2498) knots 0 0 0 0 1 1 1 1
  line L495 (142.6633, -51.2498) -> (141.896, -51.2498)
  spline S460 degree 3 poles (141.896, -51.2498) (141.8696, -51.2498) (141.896, -51.2763) (141.896, -51.2498) knots 0 0 0 0 1 1 1 1
  line L496 (141.896, -51.2498) -> (141.896, -49.7152)
  spline S461 degree 3 poles (141.896, -49.7152) (141.896, -49.6888) (141.8696, -49.7152) (141.896, -49.7152) knots 0 0 0 0 1 1 1 1
  line L497 (141.896, -49.7152) -> (142.6633, -49.7152)
  spline S462 degree 3 poles (142.6633, -49.7152) (142.6779, -49.7152) (142.6898, -49.7033) (142.6898, -49.6888) knots 0 0 0 0 1 1 1 1
  line L498 (142.6898, -49.6888) -> (142.6898, -48.1013)
  spline S463 degree 3 poles (142.6898, -48.1013) (142.6898, -48.0867) (142.6779, -48.0748) (142.6633, -48.0748) knots 0 0 0 0 1 1 1 1
  line L499 (142.6633, -48.0748) -> (141.896, -48.0748)
  spline S464 degree 3 poles (141.896, -48.0748) (141.8696, -48.0748) (141.896, -48.1013) (141.896, -48.0748) knots 0 0 0 0 1 1 1 1
  line L500 (141.896, -48.0748) -> (141.896, -46.5402)
  spline S465 degree 3 poles (141.896, -46.5402) (141.896, -46.5138) (141.8696, -46.5402) (141.896, -46.5402) knots 0 0 0 0 1 1 1 1
  line L501 (141.896, -46.5402) -> (142.6633, -46.5402)
  spline S466 degree 3 poles (142.6633, -46.5402) (142.6779, -46.5402) (142.6898, -46.5283) (142.6898, -46.5138) knots 0 0 0 0 1 1 1 1
  line L502 (142.6898, -46.5138) -> (142.6898, -44.9263)
  spline S467 degree 3 poles (142.6898, -44.9263) (142.6898, -44.9117) (142.6779, -44.8998) (142.6633, -44.8998) knots 0 0 0 0 1 1 1 1
  line L503 (142.6633, -44.8998) -> (141.896, -44.8998)
  spline S468 degree 3 poles (141.896, -44.8998) (141.8696, -44.8998) (141.896, -44.9263) (141.896, -44.8998) knots 0 0 0 0 1 1 1 1
  line L504 (141.896, -44.8998) -> (141.896, -43.3652)
  spline S469 degree 3 poles (141.896, -43.3652) (141.896, -43.3388) (141.8696, -43.3652) (141.896, -43.3652) knots 0 0 0 0 1 1 1 1
  line L505 (141.896, -43.3652) -> (142.6633, -43.3652)
  spline S470 degree 3 poles (142.6633, -43.3652) (142.6779, -43.3652) (142.6898, -43.3533) (142.6898, -43.3388) knots 0 0 0 0 1 1 1 1
  line L506 (142.6898, -43.3388) -> (142.6898, -42.545)
  spline S471 degree 3 poles (142.6898, -42.545) (142.6898, -42.5304) (142.6779, -42.5185) (142.6633, -42.5185) knots 0 0 0 0 1 1 1 1
  line L507 (142.6633, -42.5185) -> (141.8696, -42.5185)
  line L508 (141.8696, -42.5185) -> (115.4113, -42.5185)
  line L509 (115.4113, -42.5185) -> (114.6175, -42.5185)
  spline S472 degree 3 poles (114.6175, -42.5185) (114.6029, -42.5185) (114.591, -42.5304) (114.591, -42.545) knots 0 0 0 0 1 1 1 1
  line L510 (114.591, -42.545) -> (114.591, -43.3388)
  spline S473 degree 3 poles (114.591, -43.3388) (114.591, -43.3533) (114.6029, -43.3652) (114.6175, -43.3652) knots 0 0 0 0 1 1 1 1
  line L511 (114.6175, -43.3652) -> (115.3848, -43.3652)
  spline S474 degree 3 poles (115.3848, -43.3652) (115.4113, -43.3652) (115.3848, -43.3388) (115.3848, -43.3652) knots 0 0 0 0 1 1 1 1
  line L512 (115.3848, -43.3652) -> (115.3848, -44.8998)
  spline S475 degree 3 poles (115.3848, -44.8998) (115.3848, -44.9263) (115.4113, -44.8998) (115.3848, -44.8998) knots 0 0 0 0 1 1 1 1
  line L513 (115.3848, -44.8998) -> (114.6175, -44.8998)
  spline S476 degree 3 poles (114.6175, -44.8998) (114.6029, -44.8998) (114.591, -44.9117) (114.591, -44.9263) knots 0 0 0 0 1 1 1 1
  line L514 (114.591, -44.9263) -> (114.591, -46.5138)
  spline S477 degree 3 poles (114.591, -46.5138) (114.591, -46.5283) (114.6029, -46.5402) (114.6175, -46.5402) knots 0 0 0 0 1 1 1 1
  line L515 (114.6175, -46.5402) -> (115.3848, -46.5402)
  spline S478 degree 3 poles (115.3848, -46.5402) (115.4113, -46.5402) (115.3848, -46.5138) (115.3848, -46.5402) knots 0 0 0 0 1 1 1 1
  line L516 (115.3848, -46.5402) -> (115.3848, -48.0748)
  spline S479 degree 3 poles (115.3848, -48.0748) (115.3848, -48.1013) (115.4113, -48.0748) (115.3848, -48.0748) knots 0 0 0 0 1 1 1 1
  line L517 (115.3848, -48.0748) -> (114.6175, -48.0748)
  spline S480 degree 3 poles (114.6175, -48.0748) (114.6029, -48.0748) (114.591, -48.0867) (114.591, -48.1013) knots 0 0 0 0 1 1 1 1
  line L518 (114.591, -48.1013) -> (114.591, -49.6888)
  spline S481 degree 3 poles (114.591, -49.6888) (114.591, -49.7033) (114.6029, -49.7152) (114.6175, -49.7152) knots 0 0 0 0 1 1 1 1
  line L519 (114.6175, -49.7152) -> (115.3848, -49.7152)
  spline S482 degree 3 poles (115.3848, -49.7152) (115.4113, -49.7152) (115.3848, -49.6888) (115.3848, -49.7152) knots 0 0 0 0 1 1 1 1
  line L520 (115.3848, -49.7152) -> (115.3848, -51.2498)
  spline S483 degree 3 poles (115.3848, -51.2498) (115.3848, -51.2763) (115.4113, -51.2498) (115.3848, -51.2498) knots 0 0 0 0 1 1 1 1
  line L521 (115.3848, -51.2498) -> (114.6175, -51.2498)
  spline S484 degree 3 poles (114.6175, -51.2498) (114.6029, -51.2498) (114.591, -51.2617) (114.591, -51.2763) knots 0 0 0 0 1 1 1 1
  line L522 (114.591, -51.2763) -> (114.591, -52.8638)
  spline S485 degree 3 poles (114.591, -52.8638) (114.591, -52.8783) (114.6029, -52.8902) (114.6175, -52.8902) knots 0 0 0 0 1 1 1 1
  line L523 (114.6175, -52.8902) -> (115.3848, -52.8902)
  spline S486 degree 3 poles (115.3848, -52.8902) (115.4113, -52.8902) (115.3848, -52.8638) (115.3848, -52.8902) knots 0 0 0 0 1 1 1 1
  line L524 (115.3848, -52.8902) -> (115.3848, -54.4248)
  spline S487 degree 3 poles (115.3848, -54.4248) (115.3848, -54.4513) (115.4113, -54.4248) (115.3848, -54.4248) knots 0 0 0 0 1 1 1 1
  line L525 (115.3848, -54.4248) -> (114.6175, -54.4248)
  spline S488 degree 3 poles (114.6175, -54.4248) (114.6029, -54.4248) (114.591, -54.4367) (114.591, -54.4513) knots 0 0 0 0 1 1 1 1
  line L526 (114.591, -54.4513) -> (114.591, -56.0388)
  spline S489 degree 3 poles (114.591, -56.0388) (114.591, -56.0533) (114.6029, -56.0652) (114.6175, -56.0652) knots 0 0 0 0 1 1 1 1
  line L527 (114.6175, -56.0652) -> (115.3848, -56.0652)
  spline S490 degree 3 poles (115.3848, -56.0652) (115.4113, -56.0652) (115.3848, -56.0388) (115.3848, -56.0652) knots 0 0 0 0 1 1 1 1
  line L528 (115.3848, -56.0652) -> (115.3848, -57.5998)
  spline S491 degree 3 poles (115.3848, -57.5998) (115.3848, -57.6263) (115.4113, -57.5998) (115.3848, -57.5998) knots 0 0 0 0 1 1 1 1
  line L529 (115.3848, -57.5998) -> (114.6175, -57.5998)
  spline S492 degree 3 poles (114.6175, -57.5998) (114.6029, -57.5998) (114.591, -57.6117) (114.591, -57.6263) knots 0 0 0 0 1 1 1 1
  line L530 (114.591, -57.6263) -> (114.591, -58.42)
  spline S493 degree 3 poles (114.591, -58.42) (114.591, -58.4346) (114.6029, -58.4465) (114.6175, -58.4465) knots 0 0 0 0 1 1 1 1
  line L531 (114.6175, -58.4465) -> (115.4113, -58.4465)
  line L532 (143.1131, -59.2402) -> (153.6965, -59.2402)
  spline S494 degree 3 poles (153.6965, -59.2402) (153.711, -59.2402) (153.7229, -59.2283) (153.7229, -59.2138) knots 0 0 0 0 1 1 1 1
  line L533 (153.7229, -59.2138) -> (153.7229, -48.6304)
  spline S495 degree 3 poles (153.7229, -48.6304) (153.7229, -48.6257) (153.7216, -48.6212) (153.7195, -48.6172) knots 0 0 0 0 1 1 1 1
  spline S496 degree 3 poles (153.7195, -48.6172) (153.7171, -48.6132) (153.7137, -48.6098) (153.7097, -48.6074) knots 0 0 0 0 1 1 1 1
  spline S497 degree 3 poles (153.7097, -48.6074) (153.7057, -48.6053) (153.7012, -48.604) (153.6965, -48.604) knots 0 0 0 0 1 1 1 1
  spline S498 degree 3 poles (153.6965, -48.604) (153.6917, -48.604) (153.6872, -48.6053) (153.6832, -48.6074) knots 0 0 0 0 1 1 1 1
  spline S499 degree 3 poles (153.6832, -48.6074) (153.6793, -48.6098) (153.6758, -48.6132) (153.6734, -48.6172) knots 0 0 0 0 1 1 1 1
  spline S500 degree 3 poles (153.6734, -48.6172) (153.6713, -48.6212) (153.67, -48.6257) (153.67, -48.6304) knots 0 0 0 0 1 1 1 1
  spline S501 degree 3 poles (153.67, -48.6304) (153.67, -50.4836) (153.1821, -52.3039) (152.2555, -53.9089) knots 0 0 0 0 1 1 1 1
  spline S502 degree 3 poles (152.2555, -53.9089) (151.329, -55.5138) (149.9965, -56.8463) (148.3916, -57.7728) knots 0 0 0 0 1 1 1 1
  spline S503 degree 3 poles (148.3916, -57.7728) (146.7866, -58.6994) (144.9663, -59.1873) (143.1131, -59.1873) knots 0 0 0 0 1 1 1 1
  spline S504 degree 3 poles (143.1131, -59.1873) (143.1179, -59.1873) (143.1224, -59.1886) (143.1264, -59.1907) knots 0 0 0 0 1 1 1 1
  spline S505 degree 3 poles (143.1264, -59.1907) (143.1303, -59.1931) (143.1338, -59.1966) (143.1361, -59.2005) knots 0 0 0 0 1 1 1 1
  spline S506 degree 3 poles (143.1361, -59.2005) (143.1383, -59.2045) (143.1396, -59.209) (143.1396, -59.2138) knots 0 0 0 0 1 1 1 1
  spline S507 degree 3 poles (143.1396, -59.2138) (143.1396, -59.2185) (143.1383, -59.223) (143.1361, -59.227) knots 0 0 0 0 1 1 1 1
  spline S508 degree 3 poles (143.1361, -59.227) (143.1338, -59.2309) (143.1303, -59.2344) (143.1264, -59.2368) knots 0 0 0 0 1 1 1 1
  spline S509 degree 3 poles (143.1264, -59.2368) (143.1224, -59.2389) (143.1179, -59.2402) (143.1131, -59.2402) knots 0 0 0 0 1 1 1 1
  line L534 (153.6965, -48.2071) -> (143.1131, -48.2071)
  spline S510 degree 3 poles (143.1131, -48.2071) (143.0986, -48.2071) (143.0867, -48.219) (143.0867, -48.2335) knots 0 0 0 0 1 1 1 1
  line L535 (143.0867, -48.2335) -> (143.0867, -58.8169)
  spline S511 degree 3 poles (143.0867, -58.8169) (143.0867, -58.8216) (143.088, -58.8261) (143.0901, -58.8301) knots 0 0 0 0 1 1 1 1
  spline S512 degree 3 poles (143.0901, -58.8301) (143.0925, -58.8341) (143.0959, -58.8375) (143.0999, -58.8399) knots 0 0 0 0 1 1 1 1
  spline S513 degree 3 poles (143.0999, -58.8399) (143.1039, -58.842) (143.1084, -58.8433) (143.1131, -58.8433) knots 0 0 0 0 1 1 1 1
  spline S514 degree 3 poles (143.1131, -58.8433) (143.1179, -58.8433) (143.1224, -58.842) (143.1264, -58.8399) knots 0 0 0 0 1 1 1 1
  spline S515 degree 3 poles (143.1264, -58.8399) (143.1303, -58.8375) (143.1338, -58.8341) (143.1361, -58.8301) knots 0 0 0 0 1 1 1 1
  spline S516 degree 3 poles (143.1361, -58.8301) (143.1383, -58.8261) (143.1396, -58.8216) (143.1396, -58.8169) knots 0 0 0 0 1 1 1 1
  spline S517 degree 3 poles (143.1396, -58.8169) (143.1396, -56.9637) (143.6275, -55.1434) (144.554, -53.5384) knots 0 0 0 0 1 1 1 1
  spline S518 degree 3 poles (144.554, -53.5384) (145.4806, -51.9335) (146.8131, -50.601) (148.418, -49.6745) knots 0 0 0 0 1 1 1 1
  spline S519 degree 3 poles (148.418, -49.6745) (150.023, -48.7479) (151.8433, -48.26) (153.6965, -48.26) knots 0 0 0 0 1 1 1 1
  spline S520 degree 3 poles (153.6965, -48.26) (153.6917, -48.26) (153.6872, -48.2587) (153.6832, -48.2566) knots 0 0 0 0 1 1 1 1
  spline S521 degree 3 poles (153.6832, -48.2566) (153.6793, -48.2542) (153.6758, -48.2507) (153.6734, -48.2468) knots 0 0 0 0 1 1 1 1
  spline S522 degree 3 poles (153.6734, -48.2468) (153.6713, -48.2428) (153.67, -48.2383) (153.67, -48.2335) knots 0 0 0 0 1 1 1 1
  spline S523 degree 3 poles (153.67, -48.2335) (153.67, -48.2288) (153.6713, -48.2243) (153.6734, -48.2203) knots 0 0 0 0 1 1 1 1
  spline S524 degree 3 poles (153.6734, -48.2203) (153.6758, -48.2163) (153.6793, -48.2129) (153.6832, -48.2105) knots 0 0 0 0 1 1 1 1
  spline S525 degree 3 poles (153.6832, -48.2105) (153.6872, -48.2084) (153.6917, -48.2071) (153.6965, -48.2071) knots 0 0 0 0 1 1 1 1
  line L536 (156.5804, -59.2402) -> (185.6846, -59.2402)
  spline S526 degree 3 poles (185.6846, -59.2402) (187.6864, -59.2402) (189.6528, -58.7134) (191.3863, -57.7125) knots 0 0 0 0 1 1 1 1
  spline S527 degree 3 poles (191.3863, -57.7125) (193.1199, -56.7116) (194.5595, -55.272) (195.5604, -53.5384) knots 0 0 0 0 1 1 1 1
  spline S528 degree 3 poles (195.5604, -53.5384) (196.5613, -51.8049) (197.0881, -49.8385) (197.0881, -47.8367) knots 0 0 0 0 1 1 1 1
  spline S529 degree 3 poles (197.0881, -47.8367) (197.0881, -47.8221) (197.0762, -47.8102) (197.0617, -47.8102) knots 0 0 0 0 1 1 1 1
  line L537 (197.0617, -47.8102) -> (196.2679, -47.8102)
  spline S530 degree 3 poles (196.2679, -47.8102) (196.2534, -47.8102) (196.2415, -47.8221) (196.2415, -47.8367) knots 0 0 0 0 1 1 1 1
  spline S531 degree 3 poles (196.2415, -47.8367) (196.2415, -49.6898) (195.7536, -51.5101) (194.827, -53.1151) knots 0 0 0 0 1 1 1 1